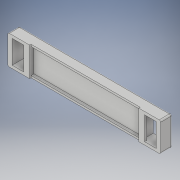
# Autodesk Inventor part: clipFemale
Saved by Autodesk Inventor 2019 (Build 230136000, 136)
## iProperties
Created: 2019-01-04
Part Number: clipFemale
Material: Generic
Document SubType Name: Modeling
Designer: Nate
Density: 1 g/cm^3
Appearance: Default
Author: Nate
Autodesk Inventor part; units mm, degrees
ref_plane "YZ Plane" through (0, 0, 0) normal (1, 0, 0) x (0, 1, 0)
ref_plane "XZ Plane" through (0, 0, 0) normal (0, 1, 0) x (-1, 0, 0)
ref_plane "XY Plane" through (0, 0, 0) normal (0, 0, 1) x (1, 0, 0)
sketch "Sketch1" plane through (0, 0, 0) normal (0, 0, 1) x (1, 0, 0)
  line L0 (0, 0) -> (66.675, 0)
  line L1 (66.675, 0) -> (66.675, 12.7)
  line L2 (66.675, 12.7) -> (0, 12.7)
  line L3 (0, 12.7) -> (0, 0)
  dimension "d0" = 66.675
  dimension "d1" = 12.7
  constraints: 8 end point, 2 parallel, 1 horizontal, 1 perpendicular
  measures "d0" distance of L2.end L1.end
  measures "d1" distance of L0.end L1.end
extrude "Extrusion1" add sketch "Sketch1" along normal blind 5.08
fillet "Fillet1" radius 0.635 4 edges at (33.3375, 12.7, 0) (66.675, 6.35, 0) (33.3375, 0, 0) (0, 6.35, 0)
fillet "Fillet2" radius 0.635 8 edges at (66.489, 12.514, 0.186) (66.675, 12.7, 2.8575) (66.489, 0.186, 0.186) (66.675, 0, 2.8575) (0.186, 12.514, 0.186) (0, 12.7, 2.8575) (0.186, 0.186, 0.186) (0, 0, 2.8575)
sketch "Sketch2" plane through (0, 0, 5.08) normal (0, 0, 1) x (1, 0, 0)
  line L0 (9.525, 12.6996) -> (57.15, 12.6996)
  line L1 (57.15, 12.6996) -> (57.15, -0.0004)
  line L2 (57.15, -0.0004) -> (9.525, -0.0004)
  line L3 (9.525, -0.0004) -> (9.525, 12.6996)
  line L4 (66.675, 0.635) -> (66.675, 12.065) projected
  point P0 (0, 0)
  dimension "d6" = 47.625
  dimension "d7" = 12.7
  dimension "d8" = 9.525
  constraints: 8 end point, 2 parallel, 1 horizontal, 1 perpendicular
  measures "d6" distance of L1.end L2.end
  measures "d7" distance of L0.end L1.end
  measures "d8" distance between parallel lines of L1 L4
extrude "Extrusion2" cut sketch "Sketch2" against normal blind 1.905
sketch "Sketch3" plane through (9.525, 12.6996, 5.08) normal (0, -1, 0) x (1, 0, 0)
  line L0 (0, -1.905) -> (0, 0) projected
  line L1 (47.625, -1.905) -> (0, -1.905) projected
  line L2 (0, 0) -> (47.625, 0)
  line L3 (47.625, 0) -> (47.625, -1.905)
  line L4 (47.625, -1.905) -> (0, -1.905)
  line L5 (0, -1.905) -> (0, 0)
  point P0 (-9.525, -5.08)
  constraints: 8 end point, 2 parallel, 1 horizontal, 1 perpendicular
extrude "Extrusion3" cut sketch "Sketch3" against normal blind 0.635
sketch "Sketch4" plane through (0, 0, 5.08) normal (0, 0, 1) x (1, 0, 0)
  line L0 (0.635, 0.635) -> (66.04, 0.635) projected
  line L1 (58.42, 11.43) -> (59.69, 11.43)
  line L2 (59.69, 11.43) -> (59.69, 1.27)
  line L3 (59.69, 1.27) -> (58.42, 1.27)
  line L4 (58.42, 1.27) -> (58.42, 11.43)
  line L5 (66.04, 12.7) -> (0.635, 12.7) projected
  line L6 (57.15, 12.7) -> (57.15, 0) projected
  line L7 (57.15, 0) -> (66.04, 0) projected
  point P0 (0, 0)
  point P1 (53.975, 6.9846)
  dimension "d13" = 1.27
  dimension "d23" = 1.27
  dimension "d24" = 1.27
  dimension "d42" = 1.27
  constraints: 8 end point, 2 parallel, 1 horizontal, 1 perpendicular, 1 other
  measures "d13" distance between parallel lines of L5 L1
  measures "d24" distance of L1.start L1.end
  measures "d42" distance from line of L7 L2.end
sketch "Sketch5" plane through (0, 0, 5.08) normal (0, 0, 1) x (1, 0, 0)
  line L0 (66.04, 12.065) -> (0.635, 12.065) projected
  line L1 (0.635, 0.635) -> (66.04, 0.635) projected
  line L2 (58.42, 11.43) -> (64.77, 11.43)
  line L3 (64.77, 11.43) -> (64.77, 1.27)
  line L4 (64.77, 1.27) -> (58.42, 1.27)
  line L5 (58.42, 1.27) -> (58.42, 11.43)
  line L6 (57.15, 12.7) -> (57.15, 0) projected
  line L7 (66.04, 12.7) -> (57.15, 12.7) projected
  line L8 (57.15, 0) -> (66.04, 0) projected
  point P0 (0, 0)
  point P1 (53.975, 6.9846)
  dimension "d14" = 6.35
  dimension "d25" = 1.27
  dimension "d43" = 1.27
  dimension "d44" = 1.27
  constraints: 8 end point, 2 parallel, 1 horizontal, 1 perpendicular, 1 other
  measures "d14" distance of L3.end L4.end
  measures "d43" distance from line of L2.end L7
  measures "d44" distance from line of L8 L3.end
extrude "Extrusion4" cut sketch "Sketch5" against normal through all
extrude "Extrusion5" add sketch "Sketch4" against normal blind 1.016
sketch "Sketch6" plane through (0, 0, 5.08) normal (0, 0, 1) x (1, 0, 0)
  line L0 (57.15, 12.7) -> (57.15, 0) projected
  line L1 (55.245, 0.635) -> (55.245, 12.065) projected
  line L2 (66.04, 12.065) -> (0.635, 12.065) projected
  line L3 (8.255, 11.43) -> (6.985, 11.43)
  line L4 (6.985, 11.43) -> (6.985, 1.27)
  line L5 (6.985, 1.27) -> (8.255, 1.27)
  line L6 (8.255, 1.27) -> (8.255, 11.43)
  line L7 (9.525, 0) -> (9.525, 12.7) projected
  line L8 (0.635, 0.635) -> (66.04, 0.635) projected
  line L9 (9.525, 12.7) -> (0.635, 12.7) projected
  line L10 (0.635, 0) -> (9.525, 0) projected
  point P0 (0, 0)
  point P1 (53.975, 6.9846)
  point P2 (6.35, 6.9846)
  dimension "d20" = 1.27
  dimension "d22" = 1.27
  dimension "d45" = 1.27
  dimension "d46" = 1.27
  constraints: 8 end point, 2 parallel, 1 horizontal, 1 perpendicular, 2 other
  measures "d20" distance of L5.end L4.end
  measures "d45" distance from line of L9 L3.end
  measures "d46" distance from line of L10 L4.end
sketch "Sketch7" plane through (0, 0, 5.08) normal (0, 0, 1) x (1, 0, 0)
  line L0 (66.04, 12.065) -> (0.635, 12.065) projected
  line L1 (8.255, 11.43) -> (1.905, 11.43)
  line L2 (1.905, 11.43) -> (1.905, 1.27)
  line L3 (1.905, 1.27) -> (8.255, 1.27)
  line L4 (8.255, 1.27) -> (8.255, 11.43)
  line L5 (9.525, 0) -> (9.525, 12.7) projected
  line L6 (0.635, 0.635) -> (66.04, 0.635) projected
  line L7 (9.525, 12.7) -> (0.635, 12.7) projected
  line L8 (0.635, 0) -> (9.525, 0) projected
  point P0 (0, 0)
  point P1 (55.245, 12.065)
  point P2 (6.35, 6.9846)
  point P3 (55.245, 0.635)
  dimension "d26" = 6.35
  dimension "d28" = 1.27
  dimension "d47" = 1.27
  dimension "d48" = 1.27
  constraints: 8 end point, 2 parallel, 1 horizontal, 1 perpendicular, 1 other
  measures "d26" distance of L3.end L2.end
  measures "d47" distance from line of L7 L1.end
  measures "d48" distance from line of L8 L2.end
extrude "Extrusion6" cut sketch "Sketch7" against normal through all
extrude "Extrusion7" add sketch "Sketch6" against normal blind 1.016 contours L6 L5 L4 L3
sketch "Sketch9" plane through (0, 0, 3.175) normal (0, 0, 1) x (1, 0, 0)
  line L0 (9.525, 0) -> (9.525, 12.7) projected
  line L1 (57.15, 12.7) -> (57.15, 0) projected
  line L2 (9.525, 12.7) -> (57.15, 12.7)
  line L3 (57.15, 12.7) -> (57.15, 11.8197)
  line L4 (57.15, 11.8197) -> (9.525, 11.8197)
  line L5 (9.525, 11.8197) -> (9.525, 12.7)
  line L6 (66.04, 0) -> (0.635, 0) projected
  line L7 (57.15, 0) -> (9.525, 0)
  line L8 (9.525, 0) -> (9.525, 0.889)
  line L9 (9.525, 0.889) -> (57.15, 0.889)
  line L10 (57.15, 0.889) -> (57.15, 0)
  point P0 (0, 0)
  point P1 (6.35, 6.9846)
  point P2 (53.975, 6.9846)
  dimension "d35" = 47.625
  dimension "d36" = 0.889
  constraints: 16 end point, 4 parallel, 2 horizontal, 2 perpendicular, 2 point on line, 3 other
  measures "d35" distance of L8.end L9.end
  measures "d36" distance of L7.end L8.end
extrude "Extrusion8" add sketch "Sketch9" along normal blind 1.27 contours L0 L9 L1 L6 | L0 L2 L1 L4
body "Solid1"
